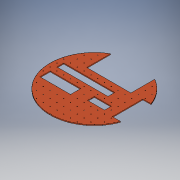
# Autodesk Inventor part: existing copper plate 2
Saved by Autodesk Inventor 2018 (Build 220112000, 112)
## iProperties
Created: 2018-11-02
Part Number: existing copper plate 2
Material: Copper
Document SubType Name: Modeling
Designer: freyja
Mass: 1508.02 g
Surface Area: 1147.68 cm^2
Volume: 168.682 cm^3
Density: 8.94 g/cm^3
Appearance: Copper - Satin
Author: freyja
Autodesk Inventor part; units mm, degrees
ref_plane "YZ Plane" through (0, 0, 0) normal (1, 0, 0) x (0, 1, 0)
ref_plane "XZ Plane" through (0, 0, 0) normal (0, 1, 0) x (-1, 0, 0)
ref_plane "XY Plane" through (0, 0, 0) normal (0, 0, 1) x (1, 0, 0)
sketch "Sketch1" plane through (0, 0, 0) normal (0, 1, 0) x (-1, 0, 0)
  circle A0 centre (0, 0) radius 165.1
  dimension "d0" = 330.2
  constraints: 1 centre point, 1 coincident
  measures "d0" diameter of A0
extrude "Extrusion1" add sketch "Sketch1" along normal blind 3.175
sketch "Sketch2" plane through (0, 3.175, 0) normal (0, 1, 0) x (1, 0, 0)
  circle A0 centre (0, 0) radius 165.1 projected
  line L0 (82.55, 142.9808) -> (82.55, 54.0808)
  line L1 (82.55, 142.9808) -> (171.45, 142.9808) construction
  line L2 (82.55, 54.0808) -> (-82.55, 54.0808)
  line L3 (-82.55, 54.0808) -> (-82.55, 142.9808)
  circle A1 centre (0, 0) radius 165.1 projected
  line L4 (82.55, 54.0808) -> (-82.55, 54.0808)
  line L5 (-82.55, 54.0808) -> (-82.55, 181.0808)
  line L6 (-82.55, 181.0808) -> (82.55, 181.0808)
  line L7 (82.55, 181.0808) -> (82.55, 54.0808)
  line L8 (-139.7, 25.5058) -> (50.8, 25.5058)
  line L9 (50.8, 25.5058) -> (50.8, 0.1058)
  line L10 (50.8, 0.1058) -> (-139.7, 0.1058)
  line L11 (-139.7, 0.1058) -> (-139.7, 25.5058)
  line L12 (-165.1, 0.1058) -> (-139.7, 0.1058) construction
  line L13 (-139.7, -63.3942) -> (-25.4, -63.3942)
  line L14 (-25.4, -63.3942) -> (-25.4, -25.2942)
  line L15 (-25.4, -25.2942) -> (-139.7, -25.2942)
  line L16 (-139.7, -25.2942) -> (-139.7, -63.3942)
  line L17 (25.4, -50.6942) -> (88.9, -50.6942)
  line L18 (88.9, -50.6942) -> (88.9, -25.2942)
  line L19 (88.9, -25.2942) -> (25.4, -25.2942)
  line L20 (25.4, -25.2942) -> (25.4, -50.6942)
  line L21 (154.8931, 57.15) -> (124.4131, 57.15) construction
  line L22 (154.8931, -57.15) -> (124.4131, -57.15) construction
  line L23 (124.4131, 57.15) -> (124.4131, -57.15) construction
  line L24 (124.4131, -57.15) -> (200.6131, -57.15)
  line L25 (200.6131, -57.15) -> (200.6131, 57.15)
  line L26 (200.6131, 57.15) -> (124.4131, 57.15)
  line L27 (124.4131, 57.15) -> (124.4131, -57.15)
  dimension "d3" = 88.9
  dimension "d4" = 90
  dimension "d5" = 165.1
  dimension "d6" = 88.9
  dimension "d7" = 90
  dimension "d8" = 127
  dimension "d10" = 190.5
  dimension "d11" = 25.4
  dimension "d12" = 25.4
  dimension "d13" = 114.3
  dimension "d14" = 38.1
  dimension "d15" = 25.4
  dimension "d16" = 28.575
  dimension "d17" = 63.5
  dimension "d18" = 25.4
  dimension "d19" = 25.4
  dimension "d20" = 50.8
  dimension "d21" = 30.48
  dimension "d22" = 30.48
  dimension "d23" = 114.3
  dimension "d24" = 76.2
  constraints: 56 end point, 11 parallel, 9 perpendicular, 8 horizontal, 6 point on circle, 3 collinear, 1 vertical
  measures "d3" distance of L0.start L0.end
  measures "d4" angle of L0 L1
  measures "d5" distance of L0.end L2.end
  measures "d6" distance of L2.end L3.end
  measures "d7" angle of L2 L3
  measures "d8" distance of L4.end L5.end
  measures "d10" distance of L10.end L9.end
  measures "d11" distance of L8.end L9.end
  measures "d12" distance of L12.start L10.end
  measures "d13" distance of L15.end L14.end
  measures "d14" distance of L14.end L13.end
  measures "d15" distance between parallel lines of L15 L10
  measures "d16" distance between parallel lines of L8 L2
  measures "d17" distance of L19.end L18.end
  measures "d18" distance of L18.end L17.end
  measures "d19" distance between parallel lines of L19 L10
  measures "d20" distance between parallel lines of L14 L20
  measures "d21" distance of L21.start L21.end
  measures "d22" distance of L22.start L22.end
  measures "d23" distance between parallel lines of L22 L21
  measures "d24" distance of L26.end L25.end
extrude "Extrusion2" cut sketch "Sketch2" against normal blind 3.175 contours L0 L2 L3 A0 | L26 L25 L24 A0 | A0 L24 L27 L26 | L8 L9 L10 L11 | L16 L15 L14 L13 | L20 L19 L18 L17
sketch "Sketch3" plane through (0, 3.175, 0) normal (0, 1, 0) x (1, 0, 0)
  line L0 (0, 0) -> (0, -12.7)
  line L1 (50.8, 0.1058) -> (-139.7, 0.1058) projected
  dimension "d27" = 12.7
  dimension "d41" = 270
  constraints: 2 end point
  measures "d27" distance of L0.start L0.end
hole "Hole1" at (0, 3.175, 12.7) direction (0, -1, 0) diameter 2.159 end through all
pattern_linear "Rectangular Pattern1" count 13 spacing 25.4 along (1, 0, 0) count 13 spacing 25.4 along (0, 0, 1) of "Hole1" first direction both ways yes second direction both ways yes
body "Solid1"
